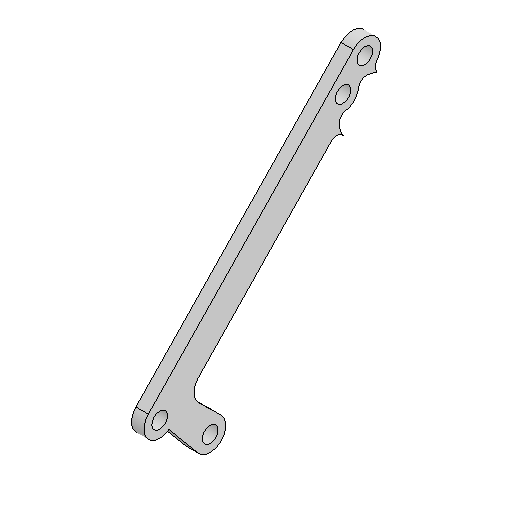
# Autodesk Inventor part: grabber arm
Saved by Autodesk Inventor 2023 (Build 270158000, 158)
## iProperties
Created: 2022-09-11
Part Number: grabber arm
Material: Generic
Document SubType Name: Modeling
Designer: deli
Density: 1 g/cm^3
Appearance: Default
Author: deli
Autodesk Inventor part; units mm, degrees
ref_plane "YZ Plane" through (0, 0, 0) normal (1, 0, 0) x (0, 1, 0)
ref_plane "XZ Plane" through (0, 0, 0) normal (0, 1, 0) x (-1, 0, 0)
ref_plane "XY Plane" through (0, 0, 0) normal (0, 0, 1) x (1, 0, 0)
sketch "Sketch1" plane through (0, 0, 0) normal (1, 0, 0) x (0, 1, 0)
  arc A0 (46.6324, -46.7557) -> (44.3932, -46.567) centre (45.3739, -48.3101) ccw projected
  line L0 (44.3932, -46.567) -> (44.0197, -46.5742) projected
  arc A1 (44.0197, -46.5742) -> (44.5828, -44.1225) centre (37.8378, -43.8639) ccw projected
  arc A2 (44.5828, -44.1225) -> (42.8512, -42.0638) centre (42.5843, -44.0459) ccw projected
  arc A3 (39.4442, -38.7851) -> (42.8512, -42.0638) centre (43.385, -38.0996) ccw projected
  arc A4 (39.4442, -38.7851) -> (37.3206, -37.1337) centre (37.4738, -39.1279) ccw projected
  arc A5 (37.3206, -37.1337) -> (34.1873, -38.1862) centre (37.8378, -43.8639) ccw projected
  arc A6 (34.1873, -38.1862) -> (34.6107, -35.1867) centre (33.1057, -36.5039) ccw projected
  arc A7 (40.3943, -29.6701) -> (34.6107, -35.1867) centre (37.6207, -32.5523) ccw construction
  line L1 (40.3943, -29.6701) -> (51.923, -40.7647) projected
  arc A8 (46.6324, -46.7557) -> (51.923, -40.7647) centre (49.1494, -43.6468) ccw projected
  arc A9 (39.4778, -31.8098) -> (38.4384, -30.7271) centre (37.6207, -32.5523) ccw construction
  arc A10 (38.4384, -30.7271) -> (39.4778, -31.8098) centre (37.6207, -32.5523) ccw construction
  arc A11 (41.5171, -37.3849) -> (42.5401, -36.2868) centre (43.385, -38.0996) ccw construction
  arc A12 (42.5401, -36.2868) -> (41.5171, -37.3849) centre (43.385, -38.0996) ccw construction
  arc A13 (49.8919, -45.5039) -> (50.9746, -44.4646) centre (49.1494, -43.6468) ccw construction
  arc A14 (50.9746, -44.4646) -> (49.8919, -45.5039) centre (49.1494, -43.6468) ccw construction
  arc A15 (45.1516, -43.7788) -> (51.923, -40.7647) centre (49.1494, -43.6468) ccw
  arc A16 (39.6467, -38.3947) -> (43.2335, -41.8465) centre (43.385, -38.0996) ccw
  arc A17 (45.1516, -43.7788) -> (43.2335, -41.8465) centre (43.1526, -43.8449) ccw
  arc A18 (39.6467, -38.3947) -> (37.6421, -36.5522) centre (37.6529, -38.5522) ccw
  arc A19 (34.6107, -35.1867) -> (37.6421, -36.5522) centre (37.6207, -32.5523) ccw
  line L2 (51.923, -40.7647) -> (-2.341, 11.4559)
  line L3 (34.847, -35.4344) -> (-0.6195, -1.3035)
  arc A20 (-2.341, 11.4559) -> (-8.344, 6.2133) centre (-5.1146, 8.5737) ccw
  circle A21 centre (49.1494, -43.6468) radius 2
  circle A22 centre (43.385, -38.0996) radius 2
  circle A23 centre (226.8258, 26.2485) radius 2
  circle A24 centre (-5.1146, 8.5737) radius 2
  line L4 (-8.344, 6.2133) -> (-17.223, -1.1957)
  arc A25 (-17.223, -1.1957) -> (-11.7999, -7.0631) centre (-14.6602, -4.2669) ccw
  line L5 (-6.2535, -1.3895) -> (-11.7999, -7.0631)
  arc A26 (-0.6195, -1.3035) -> (-6.2535, -1.3895) centre (-3.3932, -4.1857) ccw
  circle A27 centre (-14.6602, -4.2669) radius 2
  point P0 (0, 0)
  point P1 (34.6904, -35.2837)
  point P2 (51.923, -40.7647)
  dimension "d0" = 7.5
  dimension "d1" = 4
  dimension "d2" = 4
  dimension "d3" = 8
  dimension "d4" = 8
  dimension "d6" = 8
  dimension "d7" = 60
  dimension "d8" = 4
  dimension "d9" = 4
  dimension "d10" = 4
  dimension "d13" = 4
  dimension "d17" = 8
  dimension "d18" = 8
  dimension "d19" = 4
  dimension "d20" = 16
  constraints: 18 point on circle, 13 centre point, 11 tangent, 9 end point, 6 coincident, 2 concentric, 1 parallel, 1 point on line
  measures "d0" diameter of A16
  measures "d1" diameter of A17
  measures "d2" diameter of A18
  measures "d3" diameter of A19
  measures "d4" diameter of A15
  measures "d6" diameter of A20
  measures "d7" distance of L3.start L4.start
  measures "d8" diameter of A21
  measures "d9" diameter of A23
  measures "d10" diameter of A22
  measures "d13" diameter of A24
  measures "d17" diameter of A25
  measures "d18" diameter of A26
  measures "d19" diameter of A27
  measures "d20" distance of A27.centre A24.centre
extrude "Extrusion1" add sketch "Sketch1" along normal blind 3.175 contours A15 A17 A16 A18 A19 A6 L3 A26 L5 A25 L4 A20 L2 L1 A8 | A0 L0 A1 A2 A3 A4 A5 A6 L3 A19 A18 A16 A17 A15 | L3 A6 A19
equation "\"d2\" = d1"
equation "\"d3\" = d4"
equation "\"d6\" = d3"
equation "\"d9\" = d8"
equation "\"d10\" = d8"
body "Solid1"
